Autodesk Inventor part; units mm, degrees
(part 2 of 2)
  measures "d43" distance of L173.end L174.end
  measures "d44" distance of L172.end L173.end
  measures "d45" distance of L179.end L180.end
  measures "d46" distance of L178.end L179.end
  measures "d47" distance of L185.end L186.end
  measures "d48" distance of L184.end L185.end
  measures "d49" distance of L191.end L192.end
  measures "d50" distance of L190.end L191.end
  measures "d51" distance of L197.end L198.end
  measures "d52" distance of L196.end L197.end
  measures "d53" distance of L203.end L204.end
  measures "d54" distance of L202.end L203.end
  measures "d55" distance of L209.end L210.end
  measures "d56" distance of L208.end L209.end
  measures "d57" distance of L215.end L216.end
  measures "d58" distance of L214.end L215.end
  measures "d59" distance of L221.end L222.end
  measures "d60" distance of L220.end L221.end
  measures "d61" distance of L227.end L228.end
  measures "d62" distance of L226.end L227.end
  measures "d63" distance of L233.end L234.end
extrude "Extrusion1" add sketch "Sketch1" along normal blind 0.5
sketch "Sketch2" plane through (0, 0, 0.5) normal (0, 0, 1) x (1, 0, 0)
  line L0 (269.15, -107.25) -> (269.15, -87.95) projected
  line L1 (269.15, -87.95) -> (278.4, -87.95) projected
  line L2 (278.4, -87.95) -> (278.4, -64.35) projected
  line L3 (278.4, -64.35) -> (273.9, -64.35) projected
  line L4 (273.9, -64.35) -> (273.9, -42) projected
  line L5 (273.9, -42) -> (40, -42) projected
  line L6 (40, -42) -> (40, -163) projected
  line L7 (40, -163) -> (277.15, -163) projected
  line L8 (277.15, -163) -> (277.15, -145.45) projected
  line L9 (277.15, -145.45) -> (264.15, -145.45) projected
  line L10 (264.15, -145.45) -> (264.15, -126.15) projected
  line L11 (264.15, -126.15) -> (273.9, -126.15) projected
  line L12 (273.9, -126.15) -> (273.9, -107.25) projected
  line L13 (273.9, -107.25) -> (269.15, -107.25) projected
  line L14 (203, -68.25) -> (160.25, -68.25) projected
  line L15 (160.25, -68.25) -> (160.25, -61.75) projected
  line L16 (160.25, -61.75) -> (203, -61.75) projected
  line L17 (203, -61.75) -> (203, -68.25) projected
  line L18 (242.625, -146.6475) -> (244.625, -146.6475) projected
  line L19 (244.625, -146.6475) -> (244.625, -148.1475) projected
  line L20 (244.625, -148.1475) -> (246.625, -148.1475) projected
  line L21 (246.625, -148.1475) -> (246.625, -160.6475) projected
  line L22 (246.625, -160.6475) -> (240.625, -160.6475) projected
  line L23 (240.625, -160.6475) -> (240.625, -148.1475) projected
  line L24 (240.625, -148.1475) -> (242.625, -148.1475) projected
  line L25 (242.625, -148.1475) -> (242.625, -146.6475) projected
  line L26 (109.125, -146.6475) -> (111.125, -146.6475) projected
  line L27 (111.125, -146.6475) -> (111.125, -148.1475) projected
  line L28 (111.125, -148.1475) -> (113.125, -148.1475) projected
  line L29 (113.125, -148.1475) -> (113.125, -160.6475) projected
  line L30 (113.125, -160.6475) -> (107.125, -160.6475) projected
  line L31 (107.125, -160.6475) -> (107.125, -148.1475) projected
  line L32 (107.125, -148.1475) -> (109.125, -148.1475) projected
  line L33 (109.125, -148.1475) -> (109.125, -146.6475) projected
  line L34 (71, -89.3475) -> (73, -89.3475) projected
  line L35 (73, -89.3475) -> (73, -90.8475) projected
  line L36 (73, -90.8475) -> (75, -90.8475) projected
  line L37 (75, -90.8475) -> (75, -103.3475) projected
  line L38 (75, -103.3475) -> (69, -103.3475) projected
  line L39 (69, -103.3475) -> (69, -90.8475) projected
  line L40 (69, -90.8475) -> (71, -90.8475) projected
  line L41 (71, -90.8475) -> (71, -89.3475) projected
  line L42 (45, -90.8475) -> (47, -90.8475) projected
  line L43 (47, -90.8475) -> (47, -89.3475) projected
  line L44 (47, -89.3475) -> (49, -89.3475) projected
  line L45 (49, -89.3475) -> (49, -90.8475) projected
  line L46 (49, -90.8475) -> (51, -90.8475) projected
  line L47 (51, -90.8475) -> (51, -103.3475) projected
  line L48 (51, -103.3475) -> (45, -103.3475) projected
  line L49 (45, -103.3475) -> (45, -90.8475) projected
  line L50 (259.2475, -147.8975) -> (273.2525, -147.8975) projected
  line L51 (273.2525, -147.8975) -> (273.2525, -161.9025) projected
  line L52 (273.2525, -161.9025) -> (259.2475, -161.9025) projected
  line L53 (259.2475, -161.9025) -> (259.2475, -147.8975) projected
  line L54 (169.8725, -147.8975) -> (183.8775, -147.8975) projected
  line L55 (183.8775, -147.8975) -> (183.8775, -161.9025) projected
  line L56 (183.8775, -161.9025) -> (169.8725, -161.9025) projected
  line L57 (169.8725, -161.9025) -> (169.8725, -147.8975) projected
  line L58 (80.4975, -147.8975) -> (94.5025, -147.8975) projected
  line L59 (94.5025, -147.8975) -> (94.5025, -161.9025) projected
  line L60 (94.5025, -161.9025) -> (80.4975, -161.9025) projected
  line L61 (80.4975, -161.9025) -> (80.4975, -147.8975) projected
  line L62 (55.9975, -147.8975) -> (70.0025, -147.8975) projected
  line L63 (70.0025, -147.8975) -> (70.0025, -161.9025) projected
  line L64 (70.0025, -161.9025) -> (55.9975, -161.9025) projected
  line L65 (55.9975, -161.9025) -> (55.9975, -147.8975) projected
  line L66 (247.7475, -128.7975) -> (261.7525, -128.7975) projected
  line L67 (261.7525, -128.7975) -> (261.7525, -142.8025) projected
  line L68 (261.7525, -142.8025) -> (247.7475, -142.8025) projected
  line L69 (247.7475, -142.8025) -> (247.7475, -128.7975) projected
  line L70 (228.7475, -128.7975) -> (242.7525, -128.7975) projected
  line L71 (242.7525, -128.7975) -> (242.7525, -142.8025) projected
  line L72 (242.7525, -142.8025) -> (228.7475, -142.8025) projected
  line L73 (228.7475, -142.8025) -> (228.7475, -128.7975) projected
  line L74 (209.7475, -128.7975) -> (223.7525, -128.7975) projected
  line L75 (223.7525, -128.7975) -> (223.7525, -142.8025) projected
  line L76 (223.7525, -142.8025) -> (209.7475, -142.8025) projected
  line L77 (209.7475, -142.8025) -> (209.7475, -128.7975) projected
  line L78 (190.7475, -128.7975) -> (204.7525, -128.7975) projected
  line L79 (204.7525, -128.7975) -> (204.7525, -142.8025) projected
  line L80 (204.7525, -142.8025) -> (190.7475, -142.8025) projected
  line L81 (190.7475, -142.8025) -> (190.7475, -128.7975) projected
  line L82 (171.7475, -128.7975) -> (185.7525, -128.7975) projected
  line L83 (185.7525, -128.7975) -> (185.7525, -142.8025) projected
  line L84 (185.7525, -142.8025) -> (171.7475, -142.8025) projected
  line L85 (171.7475, -142.8025) -> (171.7475, -128.7975) projected
  line L86 (152.7475, -128.7975) -> (166.7525, -128.7975) projected
  line L87 (166.7525, -128.7975) -> (166.7525, -142.8025) projected
  line L88 (166.7525, -142.8025) -> (152.7475, -142.8025) projected
  line L89 (152.7475, -142.8025) -> (152.7475, -128.7975) projected
  line L90 (133.7475, -128.7975) -> (147.7525, -128.7975) projected
  line L91 (147.7525, -128.7975) -> (147.7525, -142.8025) projected
  line L92 (147.7525, -142.8025) -> (133.7475, -142.8025) projected
  line L93 (133.7475, -142.8025) -> (133.7475, -128.7975) projected
  line L94 (114.7475, -128.7975) -> (128.7525, -128.7975) projected
  line L95 (128.7525, -128.7975) -> (128.7525, -142.8025) projected
  line L96 (128.7525, -142.8025) -> (114.7475, -142.8025) projected
  line L97 (114.7475, -142.8025) -> (114.7475, -128.7975) projected
  line L98 (95.7475, -128.7975) -> (109.7525, -128.7975) projected
  line L99 (109.7525, -128.7975) -> (109.7525, -142.8025) projected
  line L100 (109.7525, -142.8025) -> (95.7475, -142.8025) projected
  line L101 (95.7475, -142.8025) -> (95.7475, -128.7975) projected
  line L102 (76.7475, -128.7975) -> (90.7525, -128.7975) projected
  line L103 (90.7525, -128.7975) -> (90.7525, -142.8025) projected
  line L104 (90.7525, -142.8025) -> (76.7475, -142.8025) projected
  line L105 (76.7475, -142.8025) -> (76.7475, -128.7975) projected
  line L106 (50.4975, -128.7975) -> (64.5025, -128.7975) projected
  line L107 (64.5025, -128.7975) -> (64.5025, -142.8025) projected
  line L108 (64.5025, -142.8025) -> (50.4975, -142.8025) projected
  line L109 (50.4975, -142.8025) -> (50.4975, -128.7975) projected
  line L110 (257.4975, -109.6975) -> (271.5025, -109.6975) projected
  line L111 (271.5025, -109.6975) -> (271.5025, -123.7025) projected
  line L112 (271.5025, -123.7025) -> (257.4975, -123.7025) projected
  line L113 (257.4975, -123.7025) -> (257.4975, -109.6975) projected
  line L114 (238.4975, -109.6975) -> (252.5025, -109.6975) projected
  line L115 (252.5025, -109.6975) -> (252.5025, -123.7025) projected
  line L116 (252.5025, -123.7025) -> (238.4975, -123.7025) projected
  line L117 (238.4975, -123.7025) -> (238.4975, -109.6975) projected
  line L118 (219.4975, -109.6975) -> (233.5025, -109.6975) projected
  line L119 (233.5025, -109.6975) -> (233.5025, -123.7025) projected
  line L120 (233.5025, -123.7025) -> (219.4975, -123.7025) projected
  line L121 (219.4975, -123.7025) -> (219.4975, -109.6975) projected
  line L122 (200.4975, -109.6975) -> (214.5025, -109.6975) projected
  line L123 (214.5025, -109.6975) -> (214.5025, -123.7025) projected
  line L124 (214.5025, -123.7025) -> (200.4975, -123.7025) projected
  line L125 (200.4975, -123.7025) -> (200.4975, -109.6975) projected
  line L126 (181.4975, -109.6975) -> (195.5025, -109.6975) projected
  line L127 (195.5025, -109.6975) -> (195.5025, -123.7025) projected
  line L128 (195.5025, -123.7025) -> (181.4975, -123.7025) projected
  line L129 (181.4975, -123.7025) -> (181.4975, -109.6975) projected
  line L130 (162.4975, -109.6975) -> (176.5025, -109.6975) projected
  line L131 (176.5025, -109.6975) -> (176.5025, -123.7025) projected
  line L132 (176.5025, -123.7025) -> (162.4975, -123.7025) projected
  line L133 (162.4975, -123.7025) -> (162.4975, -109.6975) projected
  line L134 (143.4975, -109.6975) -> (157.5025, -109.6975) projected
  line L135 (157.5025, -109.6975) -> (157.5025, -123.7025) projected
  line L136 (157.5025, -123.7025) -> (143.4975, -123.7025) projected
  line L137 (143.4975, -123.7025) -> (143.4975, -109.6975) projected
  line L138 (124.4975, -109.6975) -> (138.5025, -109.6975) projected
  line L139 (138.5025, -109.6975) -> (138.5025, -123.7025) projected
  line L140 (138.5025, -123.7025) -> (124.4975, -123.7025) projected
  line L141 (124.4975, -123.7025) -> (124.4975, -109.6975) projected
  line L142 (105.4975, -109.6975) -> (119.5025, -109.6975) projected
  line L143 (119.5025, -109.6975) -> (119.5025, -123.7025) projected
  line L144 (119.5025, -123.7025) -> (105.4975, -123.7025) projected
  line L145 (105.4975, -123.7025) -> (105.4975, -109.6975) projected
  line L146 (86.4975, -109.6975) -> (100.5025, -109.6975) projected
  line L147 (100.5025, -109.6975) -> (100.5025, -123.7025) projected
  line L148 (100.5025, -123.7025) -> (86.4975, -123.7025) projected
  line L149 (86.4975, -123.7025) -> (86.4975, -109.6975) projected
  line L150 (67.4975, -109.6975) -> (81.5025, -109.6975) projected
  line L151 (81.5025, -109.6975) -> (81.5025, -123.7025) projected
  line L152 (81.5025, -123.7025) -> (67.4975, -123.7025) projected
  line L153 (67.4975, -123.7025) -> (67.4975, -109.6975) projected
  line L154 (45.9975, -109.6975) -> (60.0025, -109.6975) projected
  line L155 (60.0025, -109.6975) -> (60.0025, -123.7025) projected
  line L156 (60.0025, -123.7025) -> (45.9975, -123.7025) projected
  line L157 (45.9975, -123.7025) -> (45.9975, -109.6975) projected
  line L158 (252.7475, -90.5975) -> (266.7525, -90.5975) projected
  line L159 (266.7525, -90.5975) -> (266.7525, -104.6025) projected
  line L160 (266.7525, -104.6025) -> (252.7475, -104.6025) projected
  line L161 (252.7475, -104.6025) -> (252.7475, -90.5975) projected
  line L162 (233.7475, -90.5975) -> (247.7525, -90.5975) projected
  line L163 (247.7525, -90.5975) -> (247.7525, -104.6025) projected
  line L164 (247.7525, -104.6025) -> (233.7475, -104.6025) projected
  line L165 (233.7475, -104.6025) -> (233.7475, -90.5975) projected
  line L166 (214.7475, -90.5975) -> (228.7525, -90.5975) projected
  line L167 (228.7525, -90.5975) -> (228.7525, -104.6025) projected
  line L168 (228.7525, -104.6025) -> (214.7475, -104.6025) projected
  line L169 (214.7475, -104.6025) -> (214.7475, -90.5975) projected
  line L170 (195.7475, -90.5975) -> (209.7525, -90.5975) projected
  line L171 (209.7525, -90.5975) -> (209.7525, -104.6025) projected
  line L172 (209.7525, -104.6025) -> (195.7475, -104.6025) projected
  line L173 (195.7475, -104.6025) -> (195.7475, -90.5975) projected
  line L174 (176.7475, -90.5975) -> (190.7525, -90.5975) projected
  line L175 (190.7525, -90.5975) -> (190.7525, -104.6025) projected
  line L176 (190.7525, -104.6025) -> (176.7475, -104.6025) projected
  line L177 (176.7475, -104.6025) -> (176.7475, -90.5975) projected
  line L178 (157.7475, -90.5975) -> (171.7525, -90.5975) projected
  line L179 (171.7525, -90.5975) -> (171.7525, -104.6025) projected
  line L180 (171.7525, -104.6025) -> (157.7475, -104.6025) projected
  line L181 (157.7475, -104.6025) -> (157.7475, -90.5975) projected
  line L182 (138.7475, -90.5975) -> (152.7525, -90.5975) projected
  line L183 (152.7525, -90.5975) -> (152.7525, -104.6025) projected
  line L184 (152.7525, -104.6025) -> (138.7475, -104.6025) projected
  line L185 (138.7475, -104.6025) -> (138.7475, -90.5975) projected
  line L186 (119.7475, -90.5975) -> (133.7525, -90.5975) projected
  line L187 (133.7525, -90.5975) -> (133.7525, -104.6025) projected
  line L188 (133.7525, -104.6025) -> (119.7475, -104.6025) projected
  line L189 (119.7475, -104.6025) -> (119.7475, -90.5975) projected
  line L190 (100.7475, -90.5975) -> (114.7525, -90.5975) projected
  line L191 (114.7525, -90.5975) -> (114.7525, -104.6025) projected
  line L192 (114.7525, -104.6025) -> (100.7475, -104.6025) projected
  line L193 (100.7475, -104.6025) -> (100.7475, -90.5975) projected
  line L194 (81.7475, -90.5975) -> (95.7525, -90.5975) projected
  line L195 (95.7525, -90.5975) -> (95.7525, -104.6025) projected
  line L196 (95.7525, -104.6025) -> (81.7475, -104.6025) projected
  line L197 (81.7475, -104.6025) -> (81.7475, -90.5975) projected
  line L198 (52.9975, -90.5975) -> (67.0025, -90.5975) projected
  line L199 (67.0025, -90.5975) -> (67.0025, -104.6025) projected
  line L200 (67.0025, -104.6025) -> (52.9975, -104.6025) projected
  line L201 (52.9975, -104.6025) -> (52.9975, -90.5975) projected
  line L202 (261.9975, -71.4975) -> (276.0025, -71.4975) projected
  line L203 (276.0025, -71.4975) -> (276.0025, -85.5025) projected
  line L204 (276.0025, -85.5025) -> (261.9975, -85.5025) projected
  line L205 (261.9975, -85.5025) -> (261.9975, -71.4975) projected
  line L206 (242.9975, -71.4975) -> (257.0025, -71.4975) projected
  line L207 (257.0025, -71.4975) -> (257.0025, -85.5025) projected
  line L208 (257.0025, -85.5025) -> (242.9975, -85.5025) projected
  line L209 (242.9975, -85.5025) -> (242.9975, -71.4975) projected
  line L210 (223.9975, -71.4975) -> (238.0025, -71.4975) projected
  line L211 (238.0025, -71.4975) -> (238.0025, -85.5025) projected
  line L212 (238.0025, -85.5025) -> (223.9975, -85.5025) projected
  line L213 (223.9975, -85.5025) -> (223.9975, -71.4975) projected
  line L214 (204.9975, -71.4975) -> (219.0025, -71.4975) projected
  line L215 (219.0025, -71.4975) -> (219.0025, -85.5025) projected
  line L216 (219.0025, -85.5025) -> (204.9975, -85.5025) projected
  line L217 (204.9975, -85.5025) -> (204.9975, -71.4975) projected
  line L218 (185.9975, -71.4975) -> (200.0025, -71.4975) projected
  line L219 (200.0025, -71.4975) -> (200.0025, -85.5025) projected
  line L220 (200.0025, -85.5025) -> (185.9975, -85.5025) projected
  line L221 (185.9975, -85.5025) -> (185.9975, -71.4975) projected
  line L222 (166.9975, -71.4975) -> (181.0025, -71.4975) projected
  line L223 (181.0025, -71.4975) -> (181.0025, -85.5025) projected
  line L224 (181.0025, -85.5025) -> (166.9975, -85.5025) projected
  line L225 (166.9975, -85.5025) -> (166.9975, -71.4975) projected
  line L226 (147.9975, -71.4975) -> (162.0025, -71.4975) projected
  line L227 (162.0025, -71.4975) -> (162.0025, -85.5025) projected
  line L228 (162.0025, -85.5025) -> (147.9975, -85.5025) projected
  line L229 (147.9975, -85.5025) -> (147.9975, -71.4975) projected
  line L230 (128.9975, -71.4975) -> (143.0025, -71.4975) projected
  line L231 (143.0025, -71.4975) -> (143.0025, -85.5025) projected
  line L232 (143.0025, -85.5025) -> (128.9975, -85.5025) projected
  line L233 (128.9975, -85.5025) -> (128.9975, -71.4975) projected
  line L234 (109.9975, -71.4975) -> (124.0025, -71.4975) projected
  line L235 (124.0025, -71.4975) -> (124.0025, -85.5025) projected
  line L236 (124.0025, -85.5025) -> (109.9975, -85.5025) projected
  line L237 (109.9975, -85.5025) -> (109.9975, -71.4975) projected
  line L238 (90.9975, -71.4975) -> (105.0025, -71.4975) projected
  line L239 (105.0025, -71.4975) -> (105.0025, -85.5025) projected
  line L240 (105.0025, -85.5025) -> (90.9975, -85.5025) projected
  line L241 (90.9975, -85.5025) -> (90.9975, -71.4975) projected
  line L242 (71.9975, -71.4975) -> (86.0025, -71.4975) projected
  line L243 (86.0025, -71.4975) -> (86.0025, -85.5025) projected
  line L244 (86.0025, -85.5025) -> (71.9975, -85.5025) projected
  line L245 (71.9975, -85.5025) -> (71.9975, -71.4975) projected
  line L246 (47.9975, -71.4975) -> (62.0025, -71.4975) projected
  line L247 (62.0025, -71.4975) -> (62.0025, -85.5025) projected
  line L248 (62.0025, -85.5025) -> (47.9975, -85.5025) projected
  line L249 (47.9975, -85.5025) -> (47.9975, -71.4975) projected
  line L250 (254.9975, -42.9975) -> (269.0025, -42.9975) projected
  line L251 (269.0025, -42.9975) -> (269.0025, -57.0025) projected
  line L252 (269.0025, -57.0025) -> (254.9975, -57.0025) projected
  line L253 (254.9975, -57.0025) -> (254.9975, -42.9975) projected
  line L254 (230.9975, -42.9975) -> (245.0025, -42.9975) projected
  line L255 (245.0025, -42.9975) -> (245.0025, -57.0025) projected
  line L256 (245.0025, -57.0025) -> (230.9975, -57.0025) projected
  line L257 (230.9975, -57.0025) -> (230.9975, -42.9975) projected
  line L258 (206.9975, -42.9975) -> (221.0025, -42.9975) projected
  line L259 (221.0025, -42.9975) -> (221.0025, -57.0025) projected
  line L260 (221.0025, -57.0025) -> (206.9975, -57.0025) projected
  line L261 (206.9975, -57.0025) -> (206.9975, -42.9975) projected
  line L262 (174.4975, -42.9975) -> (188.5025, -42.9975) projected
  line L263 (188.5025, -42.9975) -> (188.5025, -57.0025) projected
  line L264 (188.5025, -57.0025) -> (174.4975, -57.0025) projected
  line L265 (174.4975, -57.0025) -> (174.4975, -42.9975) projected
  line L266 (150.4975, -42.9975) -> (164.5025, -42.9975) projected
  line L267 (164.5025, -42.9975) -> (164.5025, -57.0025) projected
  line L268 (164.5025, -57.0025) -> (150.4975, -57.0025) projected
  line L269 (150.4975, -57.0025) -> (150.4975, -42.9975) projected
  line L270 (126.4975, -42.9975) -> (140.5025, -42.9975) projected
  line L271 (140.5025, -42.9975) -> (140.5025, -57.0025) projected
  line L272 (140.5025, -57.0025) -> (126.4975, -57.0025) projected
  line L273 (126.4975, -57.0025) -> (126.4975, -42.9975) projected
  line L274 (102.4975, -42.9975) -> (116.5025, -42.9975) projected
  line L275 (116.5025, -42.9975) -> (116.5025, -57.0025) projected
  line L276 (116.5025, -57.0025) -> (102.4975, -57.0025) projected
  line L277 (102.4975, -57.0025) -> (102.4975, -42.9975) projected
  line L278 (78.4975, -42.9975) -> (92.5025, -42.9975) projected
  line L279 (92.5025, -42.9975) -> (92.5025, -57.0025) projected
  line L280 (92.5025, -57.0025) -> (78.4975, -57.0025) projected
  line L281 (78.4975, -57.0025) -> (78.4975, -42.9975) projected
  line L282 (45.4975, -42.9975) -> (59.5025, -42.9975) projected
  line L283 (59.5025, -42.9975) -> (59.5025, -57.0025) projected
  line L284 (59.5025, -57.0025) -> (45.4975, -57.0025) projected
  line L285 (45.4975, -57.0025) -> (45.4975, -42.9975) projected
  line L286 (40, -42) -> (63.0025, -42)
  line L287 (63.0025, -42) -> (63.0025, -59.5)
  line L288 (63.0025, -59.5) -> (40, -59.5)
  line L289 (40, -59.5) -> (40, -42)
  line L290 (74.9975, -42) -> (192.0025, -42)
  line L291 (192.0025, -42) -> (192.0025, -59.5)
  line L292 (192.0025, -59.5) -> (74.9975, -59.5)
  line L293 (74.9975, -59.5) -> (74.9975, -42)
  line L294 (273.9, -42) -> (40, -42) projected
  line L295 (203.4975, -42) -> (273.9, -42)
  line L296 (273.9, -42) -> (273.9, -59.5)
  line L297 (273.9, -59.5) -> (203.4975, -59.5)
  line L298 (203.4975, -59.5) -> (203.4975, -42)
  line L299 (40, -69.5) -> (278.4, -69.5)
  point P0 (0, 0)
  dimension "d149" = 103.5
  dimension "d150" = 3.5
  dimension "d151" = 3.5
  dimension "d152" = 3.5
  dimension "d153" = 3.5
  dimension "d154" = 93.5
  constraints: 26 end point, 6 parallel, 6 point on line, 4 perpendicular, 3 horizontal, 1 collinear
  measures "d149" distance between parallel lines of L7 L288
  measures "d150" distance between parallel lines of L287 L283
  measures "d151" distance between parallel lines of L281 L293
  measures "d152" distance between parallel lines of L291 L263
  measures "d153" distance between parallel lines of L261 L298
  measures "d154" distance between parallel lines of L7 L299
extrude "Extrusion2" add sketch "Sketch2" along normal blind 2.5 contours L13 L12 L11 L10 L9 L8 L7 L6 L299 L2 L1 L0 | L6 L5 L287 L288 | L297 L298 L5 L4 | L5 L291 L292 L293
sketch "Sketch3" plane through (0, 0, 0) normal (0, 0, -1) x (-1, 0, 0)
  line L0 (-45, -88.6) -> (-45, -103.6) projected
  line L1 (-75, -103.6) -> (-75, -88.6) projected
  line L2 (-107.125, -145.9) -> (-107.125, -161.9) projected
  line L3 (-246.625, -161.9) -> (-246.625, -145.9) projected
  line L4 (-109.7525, -142.8025) -> (-95.7475, -142.8025) projected
  line L5 (-246.625, -161.9) -> (-240.625, -161.9)
  line L6 (-240.625, -161.9) -> (-240.625, -150.8975)
  line L7 (-240.625, -150.8975) -> (-113.125, -150.8975)
  line L8 (-113.125, -150.8975) -> (-113.125, -161.9)
  line L9 (-113.125, -161.9) -> (-107.125, -161.9)
  line L10 (-40, -163) -> (-277.15, -163) projected
  line L11 (-113.125, -148.1475) -> (-113.125, -160.6475) projected
  line L12 (-240.625, -160.6475) -> (-240.625, -148.1475) projected
  line L13 (-49, -90.8475) -> (-51, -90.8475) projected
  line L14 (-45, -103.6) -> (-51, -103.6)
  line L15 (-51, -103.6) -> (-51, -93.5975)
  line L16 (-51, -90.8475) -> (-51, -103.3475) projected
  line L17 (-51, -93.5975) -> (-69, -93.5975)
  line L18 (-69, -103.3475) -> (-69, -90.8475) projected
  line L19 (-69, -93.5975) -> (-69, -103.6)
  line L20 (-69, -103.6) -> (-75, -103.6)
  line L21 (-246.625, -144.8975) -> (-107.125, -144.8975)
  line L22 (-107.125, -144.8975) -> (-107.125, -145.9)
  line L23 (-246.625, -144.8975) -> (-246.625, -145.9)
  line L24 (-169.8725, -147.8975) -> (-183.8775, -147.8975) projected
  line L25 (-75, -88.6) -> (-75, -87.5975)
  line L26 (-75, -87.5975) -> (-45, -87.5975)
  line L27 (-45, -87.5975) -> (-45, -88.6)
  line L28 (-52.9975, -90.5975) -> (-67.0025, -90.5975) projected
  point P0 (0, 0)
  dimension "d172" = 3
  dimension "d173" = 3
  dimension "d174" = 3
  dimension "d175" = 3
  constraints: 32 end point, 6 perpendicular, 4 collinear, 4 point on line, 2 horizontal, 2 vertical, 1 parallel
  measures "d172" distance between parallel lines of L21 L24
  measures "d173" distance between parallel lines of L7 L24
  measures "d174" distance between parallel lines of L26 L28
  measures "d175" distance between parallel lines of L28 L17
extrude "Extrusion3" cut sketch "Sketch3" against normal blind 2
sketch "Sketch4" plane through (273.9, -126.15, 0) normal (1, 0, 0) x (0, 0, -1)
  line L0 (0, 0) -> (-3, 0) projected
  line L1 (0, 18.9) -> (-3, 18.9) projected
  line L2 (-3, 0) -> (-1.4, 0)
  line L3 (-1.4, 0) -> (-1.4, 18.9)
  line L4 (-1.4, 18.9) -> (-3, 18.9)
  line L5 (-3, 18.9) -> (-3, 0)
  point P0 (0, 126.15)
  point P1 (-1.4, 0)
  dimension "d161" = 1.6
  constraints: 8 end point, 2 parallel, 1 horizontal, 1 perpendicular, 1 point on line
  measures "d161" distance of L4.end L3.end
extrude "Extrusion4" cut sketch "Sketch4" against normal blind 2
sketch "Sketch5" plane through (278.4, -87.95, 0) normal (1, 0, 0) x (0, 0, -1)
  line L0 (-3, 0) -> (-3, 18.45) projected
  line L1 (-3, 0) -> (-1.5, 0)
  line L2 (-1.5, 0) -> (-1.5, 18.45)
  line L3 (-1.5, 18.45) -> (-3, 18.45)
  line L4 (-3, 18.45) -> (-3, 0)
  point P0 (0, 87.95)
  dimension "d164" = 1.5
  constraints: 8 end point, 2 parallel, 1 horizontal, 1 perpendicular
  measures "d164" distance of L3.end L2.end
extrude "Extrusion5" add sketch "Sketch5" along normal blind 2
sketch "Sketch6" plane through (277.15, -163, 0) normal (1, 0, 0) x (0, 0, -1)
  line L0 (0, 0) -> (-3, 0) projected
  line L1 (0, 17.55) -> (-3, 17.55) projected
  line L2 (-3, 0) -> (-1.5, 0)
  line L3 (-1.5, 0) -> (-1.5, 17.55)
  line L4 (-1.5, 17.55) -> (-3, 17.55)
  line L5 (-3, 17.55) -> (-3, 0)
  point P0 (0, 163)
  constraints: 8 end point, 2 parallel, 1 horizontal, 1 midpoint, 1 perpendicular
extrude "Extrusion6" add sketch "Sketch6" along normal blind 2
sketch "Sketch7" plane through (273.9, -64.35, 0) normal (1, 0, 0) x (0, 0, -1)
  line L0 (-0.5, 4.85) -> (-3, 4.85) projected
  line L1 (-3, 22.35) -> (-1.4, 22.35)
  line L2 (-1.4, 22.35) -> (-1.4, 4.85)
  line L3 (-1.4, 4.85) -> (-3, 4.85)
  line L4 (-3, 4.85) -> (-3, 22.35)
  point P0 (0, 64.35)
  dimension "d169" = 1.6
  constraints: 8 end point, 2 parallel, 1 horizontal, 1 perpendicular, 1 point on line
  measures "d169" distance of L2.end L3.end
extrude "Extrusion7" cut sketch "Sketch7" against normal blind 2
sketch "Sketch8" plane through (0, 0, 3) normal (0, 0, 1) x (1, 0, 0)
  line L0 (315.2975, -163) -> (253.9975, -163) construction
  line L1 (253.9975, -163) -> (253.9975, -160.05) construction
  line L2 (250.9975, -160.05) -> (253.9975, -160.05) construction
  line L3 (250.9975, -163) -> (250.9975, -160.05) construction
  line L4 (250.9975, -163) -> (234.9975, -163) construction
  line L5 (234.9975, -163) -> (234.9975, -160.05) construction
  line L6 (188.9975, -160.05) -> (234.9975, -160.05) construction
  line L7 (188.9975, -163) -> (188.9975, -160.05) construction
  line L8 (188.9975, -163) -> (163.9975, -163) construction
  line L9 (163.9975, -163) -> (163.9975, -160.05) construction
  line L10 (117.9975, -160.05) -> (163.9975, -160.05) construction
  line L11 (117.9975, -163) -> (117.9975, -160.05) construction
  line L12 (117.9975, -163) -> (77.9475, -163) construction
  line L13 (77.9475, -163) -> (77.9475, -160.05) construction
  line L14 (74.9975, -160.05) -> (77.9475, -160.05) construction
  line L15 (74.9975, -165.1) -> (74.9975, -160.05) construction
  line L16 (318.2475, -165.1) -> (74.9975, -165.1) construction
  line L17 (318.2475, -165.1) -> (318.2475, -160.05) construction
  line L18 (315.2975, -160.05) -> (318.2475, -160.05) construction
  line L19 (315.2975, -163) -> (315.2975, -160.05) construction
  line L20 (40, -163) -> (279.15, -163) projected
  line L21 (74.7975, -163) -> (78.1475, -163)
  line L22 (78.1475, -163) -> (78.1475, -159.85)
  line L23 (78.1475, -159.85) -> (74.7975, -159.85)
  line L24 (74.7975, -159.85) -> (74.7975, -163)
  line L25 (117.7975, -163) -> (164.1975, -163)
  line L26 (164.1975, -163) -> (164.1975, -159.85)
  line L27 (164.1975, -159.85) -> (117.7975, -159.85)
  line L28 (117.7975, -159.85) -> (117.7975, -163)
  line L29 (188.7975, -163) -> (235.1975, -163)
  line L30 (235.1975, -163) -> (235.1975, -159.85)
  line L31 (235.1975, -159.85) -> (188.7975, -159.85)
  line L32 (188.7975, -159.85) -> (188.7975, -163)
  line L33 (250.7975, -163) -> (254.1975, -163)
  line L34 (254.1975, -163) -> (254.1975, -159.85)
  line L35 (254.1975, -159.85) -> (250.7975, -159.85)
  line L36 (250.7975, -159.85) -> (250.7975, -163)
  line L37 (77.4475, -42) -> (189.5025, -42) construction
  line L38 (189.5025, -42) -> (189.5025, -44.95) construction
  line L39 (193.15, -44.95) -> (189.5025, -44.95) construction
  line L40 (193.15, -44.95) -> (193.15, -39.9) construction
  line L41 (74.9975, -39.9) -> (193.15, -39.9) construction
  line L42 (74.9975, -39.9) -> (74.9975, -44.95) construction
  line L43 (77.4475, -44.95) -> (74.9975, -44.95) construction
  line L44 (77.4475, -42) -> (77.4475, -44.95) construction
  line L45 (74.9975, -42) -> (77.6475, -42)
  line L46 (77.6475, -42) -> (77.6475, -45.15)
  line L47 (77.6475, -45.15) -> (74.9975, -45.15)
  line L48 (74.9975, -45.15) -> (74.9975, -42)
  line L49 (192.0025, -42) -> (74.9975, -42) projected
  line L50 (192.0025, -59.5) -> (192.0025, -42) projected
  line L51 (189.3025, -42) -> (192.0025, -42)
  line L52 (192.0025, -42) -> (192.0025, -45.15)
  line L53 (192.0025, -45.15) -> (189.3025, -45.15)
  line L54 (189.3025, -45.15) -> (189.3025, -42)
  line L55 (205.9975, -42) -> (247.7, -42) construction
  line L56 (247.7, -42) -> (247.7, -44.95) construction
  line L57 (252.4, -44.95) -> (247.7, -44.95) construction
  line L58 (252.4, -42) -> (252.4, -44.95) construction
  line L59 (252.4, -42) -> (318.0525, -42) construction
  line L60 (318.0525, -42) -> (318.0525, -44.95) construction
  line L61 (320.5025, -44.95) -> (318.0525, -44.95) construction
  line L62 (320.5025, -39.9) -> (320.5025, -44.95) construction
  line L63 (202.35, -39.9) -> (320.5025, -39.9) construction
  line L64 (202.35, -39.9) -> (202.35, -44.95) construction
  line L65 (205.9975, -44.95) -> (202.35, -44.95) construction
  line L66 (205.9975, -42) -> (205.9975, -44.95) construction
  line L67 (203.4975, -59.5) -> (203.4975, -42) projected
  line L68 (206.1975, -42) -> (203.4975, -42)
  line L69 (203.4975, -42) -> (203.4975, -45.15)
  line L70 (203.4975, -45.15) -> (206.1975, -45.15)
  line L71 (206.1975, -45.15) -> (206.1975, -42)
  line L72 (273.9, -42) -> (40, -42) projected
  line L73 (247.5, -42) -> (252.6, -42)
  line L74 (252.6, -42) -> (252.6, -45.15)
  line L75 (252.6, -45.15) -> (247.5, -45.15)
  line L76 (247.5, -45.15) -> (247.5, -42)
  point P0 (0, 0)
  dimension "d178" = 0.2
  dimension "d179" = 0.2
  dimension "d180" = 0.2
  dimension "d181" = 0.2
  dimension "d182" = 0.2
  dimension "d183" = 0.2
  dimension "d184" = 0.2
  dimension "d185" = 0.2
  dimension "d186" = 0.2
  dimension "d187" = 0.2
  dimension "d188" = 0.2
  dimension "d189" = 0.2
  dimension "d190" = 0.2
  dimension "d191" = 0.2
  dimension "d192" = 0.2
  constraints: 64 end point, 16 parallel, 8 horizontal, 8 perpendicular, 7 point on line, 4 collinear, 7 other
  measures "d178" distance between parallel lines of L23 L14
  measures "d179" distance between parallel lines of L15 L24
  measures "d180" distance between parallel lines of L22 L13
  measures "d181" distance between parallel lines of L11 L28
  measures "d182" distance between parallel lines of L26 L9
  measures "d183" distance between parallel lines of L7 L32
  measures "d184" distance between parallel lines of L30 L5
  measures "d185" distance between parallel lines of L3 L36
  measures "d186" distance between parallel lines of L34 L1
  measures "d187" distance between parallel lines of L47 L43
  measures "d188" distance between parallel lines of L46 L44
  measures "d189" distance between parallel lines of L38 L54
  measures "d190" distance between parallel lines of L71 L66
  measures "d191" distance between parallel lines of L56 L76
  measures "d192" distance between parallel lines of L74 L58
extrude "Extrusion8" cut sketch "Sketch8" against normal blind 2.5
sketch "Sketch9" plane through (0, 0, 3) normal (0, 0, 1) x (1, 0, 0)
  line L0 (231.666, -151.79) -> (236.3566, -151.79) construction
  line L1 (236.3566, -151.79) -> (236.3566, -154.838) construction
  line L2 (236.3566, -154.838) -> (231.666, -154.838) construction
  line L3 (231.666, -154.838) -> (231.666, -151.79) construction
  line L4 (232.1424, -156.79) -> (232.1424, -151.79)
  line L5 (232.1424, -151.79) -> (233.1523, -151.79)
  line L6 (233.1523, -151.79) -> (233.1523, -156.79)
  line L7 (233.1523, -156.79) -> (232.1424, -156.79)
  line L8 (235.3932, -156.79) -> (233.6058, -151.79)
  line L9 (233.6058, -151.79) -> (234.6996, -151.79)
  line L10 (234.6996, -151.79) -> (235.9686, -155.4904)
  line L11 (235.9686, -155.4904) -> (237.192, -151.79)
  line L12 (237.192, -151.79) -> (238.2628, -151.79)
  line L13 (238.2628, -151.79) -> (236.4755, -156.79)
  line L14 (236.4755, -156.79) -> (235.3932, -156.79)
  point P0 (0, 0)
  constraints: 2 other
extrude "Extrusion9" cut sketch "Sketch9" against normal blind 1
sketch "Sketch10" plane through (0, 0, 3) normal (0, 0, 1) x (1, 0, 0)
  line L0 (40, -69.5) -> (40, -163) construction
  line L1 (40, -163) -> (74.7975, -163) construction
  line L2 (40, -163) -> (277.15, -163) projected
  line L3 (40, -163) -> (50, -163)
  line L4 (50, -163) -> (50, -145)
  line L5 (50, -145) -> (40, -145)
  line L6 (40, -145) -> (40, -163)
  point P0 (0, 0)
  dimension "d197" = 10
  dimension "d198" = 18
  constraints: 8 end point, 2 parallel, 1 horizontal, 1 perpendicular
  measures "d197" distance of L4.end L5.end
  measures "d198" distance of L3.end L4.end
extrude "Extrusion10" cut sketch "Sketch10" against normal blind 3
equation "\"d0\" = gap"
equation "\"d1\" = d0"
equation "\"d2\" = d0"
equation "\"d3\" = d0"
equation "\"d4\" = d0"
equation "\"d5\" = d0"
equation "\"d6\" = d0"
equation "\"d7\" = d0"
equation "\"d8\" = d0"
equation "\"d9\" = d0"
equation "\"d10\" = d0"
equation "\"d11\" = sw"
equation "\"d12\" = sw"
equation "\"d13\" = sw"
equation "\"d14\" = sw"
equation "\"d15\" = sw"
equation "\"d16\" = sw"
equation "\"d17\" = sw"
equation "\"d18\" = sw"
equation "\"d19\" = sw"
equation "\"d20\" = sw"
equation "\"d21\" = sw"
equation "\"d22\" = sw"
equation "\"d23\" = sw"
equation "\"d24\" = sw"
equation "\"d25\" = sw"
equation "\"d26\" = sw"
equation "\"d27\" = sw"
equation "\"d28\" = sw"
equation "\"d29\" = sw"
equation "\"d30\" = sw"
equation "\"d31\" = sw"
equation "\"d32\" = sw"
equation "\"d33\" = sw"
equation "\"d34\" = sw"
equation "\"d35\" = sw"
equation "\"d36\" = sw"
equation "\"d37\" = sw"
equation "\"d38\" = sw"
equation "\"d39\" = sw"
equation "\"d40\" = sw"
equation "\"d41\" = sw"
equation "\"d42\" = sw"
equation "\"d43\" = sw"
equation "\"d44\" = sw"
equation "\"d45\" = sw"
equation "\"d46\" = sw"
equation "\"d47\" = sw"
equation "\"d48\" = sw"
equation "\"d49\" = sw"
equation "\"d50\" = sw"
equation "\"d51\" = sw"
equation "\"d52\" = sw"
equation "\"d53\" = sw"
equation "\"d54\" = sw"
equation "\"d55\" = sw"
equation "\"d56\" = sw"
equation "\"d57\" = sw"
equation "\"d58\" = sw"
equation "\"d59\" = sw"
equation "\"d60\" = sw"
equation "\"d61\" = sw"
equation "\"d62\" = sw"
equation "\"d63\" = sw"
equation "\"gap\" = 0.1"
equation "\"sw\" = 14.005"
body "Solid1"
